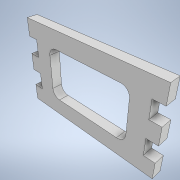
# Autodesk Inventor part: FRONT V2
Saved by Autodesk Inventor 2021.2 (Build 252289000, 289)
## iProperties
Created: 2021-03-11
Part Number: FRONT V2
Material: Generic
Document SubType Name: Modeling
Designer: 443201246
Density: 1 g/cm^3
Appearance: Default
Author: 443201246
Autodesk Inventor part; units mm, degrees
ref_plane "YZ Plane" through (0, 0, 0) normal (1, 0, 0) x (0, 1, 0)
ref_plane "XZ Plane" through (0, 0, 0) normal (0, 1, 0) x (-1, 0, 0)
ref_plane "XY Plane" through (0, 0, 0) normal (0, 0, 1) x (1, 0, 0)
sketch "Sketch1" plane through (0, 0, 0) normal (0, 0, 1) x (1, 0, 0)
  line L0 (-82, -50) -> (82, -50)
  line L1 (82, -50) -> (82, 50)
  line L2 (82, 50) -> (-82, 50)
  line L3 (-82, 50) -> (-82, -50)
  line L4 (-82, -50) -> (82, 50) construction
  line L5 (82, -50) -> (-82, 50) construction
  point P0 (0, 0)
  dimension "d0" = 164
  dimension "d1" = 100
  constraints: 12 end point, 2 midpoint, 2 parallel, 1 horizontal, 1 perpendicular
  measures "d0" distance of L2.end L1.end
  measures "d1" distance of L1.end L0.end
extrude "Extrusion1" add sketch "Sketch1" along normal mid plane 12
sketch "Sketch2" plane through (0, 0, 6) normal (0, 0, 1) x (1, 0, 0)
  line L0 (-82, 50) -> (-82, -50) projected
  line L1 (-82, -30) -> (-70, -30)
  line L2 (-70, -30) -> (-70, -10)
  line L3 (-70, -10) -> (-82, -10)
  line L4 (-82, -10) -> (-82, -30)
  line L5 (-82, -50) -> (82, -50) projected
  line L6 (-82, 10) -> (-70, 10)
  line L7 (-70, 10) -> (-70, 30)
  line L8 (-70, 30) -> (-82, 30)
  line L9 (-82, 30) -> (-82, 10)
  point P0 (0, 0)
  dimension "d4" = 12
  dimension "d5" = 20
  dimension "d6" = 20
  dimension "d7" = 20
  dimension "d8" = 20
  constraints: 16 end point, 4 parallel, 2 horizontal, 2 perpendicular, 2 point on line
  measures "d4" distance of L3.end L2.end
  measures "d5" distance of L2.end L1.end
  measures "d6" distance between parallel lines of L5 L1
  measures "d7" distance of L7.end L6.end
  measures "d8" distance between parallel lines of L6 L3
extrude "Extrusion2" cut sketch "Sketch2" against normal through all
mirror "Mirror1" about plane through (0, 0, 0) normal (1, 0, 0) of "Extrusion2"
sketch "Sketch3" plane through (0, 0, 6) normal (0, 0, 1) x (1, 0, 0)
  line L0 (-40, -30) -> (40, -30)
  line L1 (50, -20) -> (50, 20)
  line L2 (40, 30) -> (-40, 30)
  line L3 (-50, 20) -> (-50, -20)
  line L4 (-50, -30) -> (50, 30) construction
  line L5 (50, -30) -> (-50, 30) construction
  arc A0 (-40, 30) -> (-50, 20) centre (-40, 20) ccw
  arc A1 (50, 20) -> (40, 30) centre (40, 20) ccw
  arc A2 (40, -30) -> (50, -20) centre (40, -20) ccw
  arc A3 (-50, -20) -> (-40, -30) centre (-40, -20) ccw
  point P0 (0, 0)
  dimension "d11" = 100
  dimension "d12" = 60
  dimension "d13" = 10
  dimension "d14" = 10
  constraints: 12 end point, 8 point on circle, 8 point on line, 8 tangent, 4 centre point, 2 equal radius, 2 midpoint, 2 parallel, 1 horizontal, 1 perpendicular
  measures "d11" distance of L5.end L4.end
  measures "d12" distance of L4.end L5.start
  measures "d13" radius of A0
  measures "d14" radius of A1
extrude "Extrusion3" cut sketch "Sketch3" against normal through all
body "Solid1"
